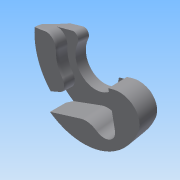
# Autodesk Inventor part: pulley_protector
Saved by Autodesk Inventor 2015 (Build 190159000, 159)
## iProperties
Created: 2014-11-28
Part Number: pulley_protector
Material: Generic
Document SubType Name: Modeling
Designer: brent
Density: 1 g/cm^3
Appearance: Default
Author: brent
Autodesk Inventor part; units mm, degrees
ref_plane "YZ Plane" through (0, 0, 0) normal (1, 0, 0) x (0, 1, 0)
ref_plane "XZ Plane" through (0, 0, 0) normal (0, 1, 0) x (-1, 0, 0)
ref_plane "XY Plane" through (0, 0, 0) normal (0, 0, 1) x (1, 0, 0)
derived "mount_alt.ipt"
sketch "Sketch15" plane through (-81.0846, 18.0799, 0) normal (0, 0, -1) x (-0.9721651, -0.2342969, 0)
  arc A0 (-39.3871, 15.0247) -> (-10.4511, 23.2872) centre (-59.5437, 140.415) ccw
  arc A1 (-0.6905, 25.25) -> (-10.4511, 23.2872) centre (-0.6905, 0) ccw
  line L0 (-0.6905, 25.25) -> (0.6905, 25.25)
  arc A2 (0.6905, -25.25) -> (0.6905, 25.25) centre (0.6905, 0) ccw
  line L1 (0.6905, -25.25) -> (-0.6905, -25.25)
  arc A3 (-10.4511, -23.2872) -> (-0.6905, -25.25) centre (-0.6905, 0) ccw
  arc A4 (-10.4511, -23.2872) -> (-39.3871, -15.0247) centre (-59.5437, -140.415) ccw
  arc A5 (-44.3006, -6.4617) -> (-39.3871, -15.0247) centre (-38.3792, -8.7552) ccw
  arc A6 (-44.3006, -6.4617) -> (-44.3006, 6.4617) centre (-60.9829, 0) ccw
  arc A7 (-39.3871, 15.0247) -> (-44.3006, 6.4617) centre (-38.3792, 8.7552) ccw
  arc A8 (-78.7459, 18.486) -> (-79.5079, 17.724) centre (-78.7459, 17.724) ccw
  line L2 (-79.5079, 0.7938) -> (-79.5079, 17.724)
  line L3 (-69.9478, 0.7938) -> (-79.5079, 0.7938)
  arc A9 (-69.9478, -0.7937) -> (-69.9478, 0.7938) centre (-60.9829, 0) ccw
  line L4 (-79.5079, -0.7937) -> (-69.9478, -0.7937)
  line L5 (-79.5079, -17.7803) -> (-79.5079, -0.7937)
  arc A10 (-79.5079, -17.7803) -> (-78.7459, -18.5423) centre (-78.7459, -17.7803) ccw
  line L6 (-67.4226, -18.5423) -> (-78.7459, -18.5423)
  arc A11 (-65.4775, -18.6922) -> (-67.4226, -18.5423) centre (-67.4226, -31.2423) ccw
  line L7 (-4.365, -28.1637) -> (-65.4775, -18.6922)
  arc A12 (-4.365, -28.1637) -> (-4.365, 28.1637) centre (0, 0) ccw
  line L8 (-65.8411, 18.6358) -> (-4.365, 28.1637)
  arc A13 (-67.7862, 18.486) -> (-65.8411, 18.6358) centre (-67.7862, 31.186) ccw
  line L9 (-78.7459, 18.486) -> (-67.7862, 18.486)
  arc A14 (-44.3006, -6.4617) -> (-39.3871, -15.0247) centre (-38.3792, -8.7552) ccw
  arc A15 (-10.4511, -23.2872) -> (-39.3871, -15.0247) centre (-59.5437, -140.415) ccw
  arc A16 (-10.4511, 23.2872) -> (-10.4511, -23.2872) centre (-0.6905, 0) ccw
  arc A17 (-39.3871, 15.0247) -> (-10.4511, 23.2872) centre (-59.5437, 140.415) ccw
  arc A18 (-39.3871, 15.0247) -> (-44.3006, 6.4617) centre (-38.3792, 8.7552) ccw
  arc A19 (-44.3006, -6.4617) -> (-44.3006, 6.4617) centre (-60.9829, 0) ccw
  point P0 (-74.5915, -36.5745)
derived "mount_sketch_alt.ipt"
sketch "Sketch2" plane through (0, 0, 0) normal (0, 0, 1) x (1, 0, 0)
  line L0 (0.3761, 19.4229) -> (-3.6038, 35.9366) projected
  line L1 (-11.1943, 15.8506) -> (-0.1862, 18.5036) projected
  line L2 (-70.2424, -8.2772) -> (-13.0502, 15.2492) projected
  arc A0 (-11.1943, 15.8506) -> (-13.0502, 15.2492) centre (-8.2187, 3.5041) ccw projected
  arc A1 (-39.2736, 12.7016) -> (-65.4683, -2.1105) centre (9.7006, -104.4757) ccw projected
  arc A2 (-39.2736, 12.7016) -> (-36.5032, 22.1775) centre (-41.7223, 18.5605) ccw projected
  arc A3 (-39.531, 34.7412) -> (-36.5032, 22.1775) centre (-21.7992, 32.368) ccw projected
  line L3 (-3.9758, 37.48) -> (-7.9425, 53.9389) projected
  line L4 (-8.8618, 54.5012) -> (-19.5164, 51.9334) projected
  arc A4 (-46.1419, 9.5883) -> (-39.742, 4.2693) centre (-21.7992, 32.368) ccw
  line L5 (-13.2697, 35.2401) -> (-3.9758, 37.48) projected
  line L6 (-3.6038, 35.9366) -> (-12.8978, 33.6968) projected
  circle A5 centre (-21.7992, 32.368) radius 12.5
  line L7 (-9.4856, 34.5191) -> (10.7885, 39.4053)
  arc A6 (-39.531, 34.7412) -> (-46.3141, 41.9146) centre (-45.8249, 35.5835) ccw projected
  arc A7 (-76.3805, 43.1675) -> (-46.3141, 41.9146) centre (-56.097, 168.5373) ccw projected
  arc A8 (-39.531, 34.7412) -> (-36.5032, 22.1775) centre (-21.7992, 32.368) ccw projected
  line L8 (-46.3141, 41.9146) -> (-23.3423, 44.7723)
  arc A9 (-53.8466, 41.5572) -> (-46.1419, 9.5883) centre (-21.7992, 32.368) ccw
  arc A10 (-39.742, 4.2693) -> (10.7885, 39.4053) centre (-21.7992, 32.368) ccw
  arc A11 (10.7885, 39.4053) -> (-53.8466, 41.5572) centre (-21.7992, 32.368) ccw
  line L9 (-0.1862, 18.5036) -> (0.5546, 18.6821)
  line L10 (0.5546, 18.6821) -> (0.3761, 19.4229)
  point P0 (0, 0)
  dimension "d2" = 66.6778
  dimension "d3" = 25
  constraints: 13 point on circle, 8 end point, 5 centre point, 2 coincident, 2 point on line, 1 parallel, 1 tangent
  measures "d2" diameter of A4
  measures "d3" diameter of A5
extrude "Extrusion1" add sketch "Sketch2" along normal blind 6.35 contours L10 L9 L1 A0 L2 A4 A1 A2 A3 A6 L8 A5 L6 L0 | L0 L7 A10 L2 A0 L1 L9 L10 | A7 A6 A3 A2 A1 A9
extrude "Extrusion2" add sketch "Sketch2" against normal blind 6.35 contours A7 A6 A3 A2 A1 A9
extrude "Extrusion3" add sketch "Sketch2" against normal blind 12.7 contours L0 L7 A10 L2 A0 L1 L9 L10
fillet "Fillet1" radius 3.175 1 edges at (-23.3423, 44.7723, 3.175)
chamfer "Chamfer1" distance 0.254 angle 45 5 edges at (-41.211, 39.9463, -6.35) (-39.1912, 28.1764, -6.35) (-35.6274, 16.7786, -6.35) (-42.7309, 11.196, -6.35) (-50.0777, 41.68, -6.35)
fillet "Fillet2" radius 5.08 5 edges at (-35.6274, 16.7786, -6.096) (-42.7309, 11.196, -6.096) (-41.211, 39.9463, -6.096) (-50.0777, 41.68, -6.096) (-39.1912, 28.1764, -6.096)
fillet "Fillet3" radius 9.8425 1 edges at (10.7885, 39.4053, -3.175)
chamfer "Chamfer2" distance 8.89 angle 45 3 edges at (-30.2493, 0.1177, 6.35) (8.0093, 33.9075, 6.35) (-5.3654, 35.5121, 6.35)
sketch "Sketch3" plane through (0, 0, -12.7) normal (0, 0, -1) x (-1, 0, 0)
  line L0 (-0.5546, 18.6821) -> (11.1943, 15.8506) projected
  circle A0 centre (5.3198, 17.2663) radius 6.0427
  point P0 (0, 0)
  constraints: 1 midpoint, 3 other
extrude "Extrusion4" cut sketch "Sketch3" against normal up to surface (12.7 mm away)
fillet "Fillet4" radius 9.8425 1 edges at (-11.1943, 15.8506, -6.35)
mirror "Mirror1" about plane through (-45.863, 26.5684, 6.35) normal (0, 0, 1) remove original yes
body "Solid1"
